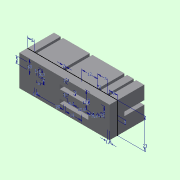
# Autodesk Inventor part: Spirulina_prototype
Saved by Autodesk Inventor 2015 (Build 190159000, 159)
## iProperties
Created: 2015-05-18
Part Number: Spirulina_prototype
Material: Generic
Document SubType Name: Modeling
Designer: Openlab
Density: 1 g/cm^3
Appearance: Default
Author: Openlab
Autodesk Inventor part; units mm, degrees
ref_plane "YZ Plane" through (0, 0, 0) normal (1, 0, 0) x (0, 1, 0)
ref_plane "XZ Plane" through (0, 0, 0) normal (0, 1, 0) x (-1, 0, 0)
ref_plane "XY Plane" through (0, 0, 0) normal (0, 0, 1) x (1, 0, 0)
sketch "Sketch1" plane through (0, 0, 0) normal (0, 1, 0) x (-1, 0, 0)
  line L0 (73.3629, -5.9836) -> (60.8629, -5.9836)
  line L1 (60.8629, -5.9836) -> (60.8629, -18.4836)
  line L2 (60.8629, -18.4836) -> (73.3629, -18.4836)
  line L3 (73.3629, -18.4836) -> (73.3629, -5.9836)
  line L4 (107.9129, -0.7336) -> (40.3129, -0.7336)
  line L5 (40.3129, -23.7336) -> (107.9129, -23.7336)
  line L6 (77.3838, -12.2336) -> (49.3838, -12.2336) construction
  line L7 (67.1129, -2.25) -> (67.1129, -23.25) construction
  line L8 (81.1129, -9.7336) -> (107.9129, -9.7336)
  line L9 (107.9129, -14.7336) -> (81.1129, -14.7336)
  line L10 (48.1129, -23.7336) -> (48.1129, -0.7336)
  line L11 (46.3129, -0.7336) -> (46.3129, -23.7336)
  line L12 (52.6129, -10.7336) -> (40.3129, -10.7336)
  line L13 (52.6129, -13.7336) -> (40.3129, -13.7336)
  line L14 (101.1129, -15.2836) -> (99.6129, -15.2836)
  line L15 (99.6129, -15.2836) -> (99.6129, -9.1836)
  line L16 (99.6129, -9.1836) -> (101.1129, -9.1836)
  line L17 (79.1129, -0.7336) -> (79.1129, -23.7336)
  line L18 (81.1129, -23.7336) -> (81.1129, -0.7336)
  line L19 (55.1129, -0.7336) -> (55.1129, -23.7336)
  line L20 (79.1129, -13.7336) -> (73.3629, -13.7336)
  line L21 (73.3629, -10.7336) -> (79.1129, -10.7336)
  line L22 (60.8629, -13.7336) -> (55.1129, -13.7336)
  line L23 (55.1129, -10.7336) -> (60.8629, -10.7336)
  line L24 (73.3629, -18.4836) -> (77.5629, -18.4836)
  line L25 (77.5629, -18.4836) -> (77.5629, -15.2836)
  line L26 (77.5629, -15.2836) -> (73.3629, -15.2836)
  line L27 (73.3629, -15.2836) -> (60.8629, -15.2836)
  line L28 (56.2629, -15.2836) -> (56.2629, -18.4836)
  line L29 (56.2629, -18.4836) -> (59.4629, -18.4836)
  line L30 (59.4629, -15.2836) -> (56.2629, -15.2836)
  line L31 (59.4629, -5.9836) -> (56.2629, -5.9836)
  line L32 (56.2629, -5.9836) -> (56.2629, -9.1836)
  line L33 (56.2629, -9.1836) -> (59.4629, -9.1836)
  line L34 (60.8629, -9.1836) -> (73.3629, -9.1836)
  line L35 (77.5629, -9.1836) -> (77.5629, -5.9836)
  line L36 (73.3629, -5.9836) -> (77.5629, -5.9836)
  line L37 (77.5629, -9.1836) -> (73.3629, -9.1836)
  line L38 (59.4629, -18.4836) -> (59.4629, -15.2836)
  line L39 (59.4629, -9.1836) -> (59.4629, -5.9836)
  line L40 (60.8629, -18.4836) -> (59.4629, -18.4836)
  line L41 (60.8629, -15.2836) -> (59.4629, -15.2836)
  line L42 (60.8629, -9.1836) -> (59.4629, -9.1836)
  line L43 (60.8629, -5.9836) -> (59.4629, -5.9836)
  line L44 (40.3129, -23.7336) -> (40.3129, -0.7336)
  line L45 (107.9129, -23.7336) -> (107.9129, -0.7336)
  line L46 (53.1129, -14.7336) -> (52.6129, -14.7336)
  line L47 (52.6129, -14.7336) -> (52.6129, -9.7336)
  line L48 (52.6129, -9.7336) -> (53.1129, -9.7336)
  line L49 (53.1129, -23.7336) -> (53.1129, -14.7336)
  line L50 (53.1129, -9.7336) -> (53.1129, -0.7336)
  line L51 (101.1129, -16.2336) -> (98.1129, -16.2336)
  line L52 (98.1129, -16.2336) -> (98.1129, -18.2336)
  line L53 (98.1129, -18.2336) -> (101.1129, -18.2336)
  line L54 (102.9129, -16.2336) -> (105.9129, -16.2336)
  line L55 (105.9129, -16.2336) -> (105.9129, -18.2336)
  line L56 (105.9129, -18.2336) -> (102.9129, -18.2336)
  line L57 (101.1129, -8.2336) -> (98.1129, -8.2336)
  line L58 (98.1129, -8.2336) -> (98.1129, -6.2336)
  line L59 (98.1129, -6.2336) -> (101.1129, -6.2336)
  line L60 (102.9129, -8.2336) -> (105.9129, -8.2336)
  line L61 (105.9129, -8.2336) -> (105.9129, -6.2336)
  line L62 (105.9129, -6.2336) -> (102.9129, -6.2336)
  line L63 (106.4404, -17.2336) -> (97.7013, -17.2336) construction
  line L64 (106, -7.2336) -> (98, -7.2336) construction
  line L65 (102.9129, -23.7336) -> (102.9129, -18.2336)
  line L66 (101.1129, -18.2336) -> (101.1129, -23.7336)
  line L67 (102.9129, -16.2336) -> (102.9129, -8.2336)
  line L68 (102.9129, -6.2336) -> (102.9129, -0.7336)
  line L69 (101.1129, -0.7336) -> (101.1129, -6.2336)
  line L70 (101.1129, -8.2336) -> (101.1129, -16.2336)
  point P0 (102.9129, -9.7336)
  point P1 (101.1129, -9.7336)
  point P2 (102.9129, -14.7336)
  point P3 (101.1129, -14.7336)
  point P4 (48.1129, -10.7336)
  point P5 (46.3129, -10.7336)
  point P6 (48.1129, -13.7336)
  point P7 (46.3129, -13.7336)
  point P8 (67.1129, -12.2336)
  point P9 (99.6129, -9.7336)
  point P10 (99.6129, -14.7336)
  dimension "d0" = 12.5
  dimension "d1" = 12.5
  dimension "d12" = 5
  dimension "d18" = 1.8
  dimension "d39" = 1.5
  dimension "d43" = 2
  dimension "d52" = 12
  dimension "d57" = 12
  dimension "d62" = 3
  dimension "d63" = 3
  dimension "d71" = 7
  dimension "d76" = 4.2
  dimension "d77" = 3.2
  dimension "d78" = 3.2
  dimension "d79" = 1.4
  dimension "d80" = 3.2
  dimension "d91" = 6
  dimension "d92" = 3
  dimension "d95" = 23
  dimension "d98" = 5
  dimension "d99" = 0.5
  dimension "d100" = 2
  dimension "d101" = 2
  dimension "d102" = 3
  dimension "d103" = 10
  dimension "d104" = 1.8
  dimension "d105" = 20
  dimension "d107" = 6.1
  dimension "d108" = 5
  constraints: 138 end point, 56 point on line, 35 perpendicular, 16 vertical, 15 horizontal, 9 collinear, 8 parallel, 4 equal length, 33 other
  measures "d0" distance of L2.end L1.end
  measures "d1" distance of L0.end L1.end
  measures "d12" distance between parallel lines of L9 L8
  measures "d18" distance between parallel lines of L11 L10
  measures "d39" distance of L14.start L14.end
  measures "d43" distance between parallel lines of L18 L17
  measures "d52" distance between parallel lines of L19 L7
  measures "d57" distance between parallel lines of L17 L7
  measures "d62" distance between parallel lines of L21 L20
  measures "d63" distance between parallel lines of L23 L22
  measures "d71" distance between parallel lines of L10 L19
  measures "d76" distance of L2.end L24.end
  measures "d77" distance of L24.end L25.end
  measures "d78" distance of L35.start L35.end
  measures "d79" distance between parallel lines of L38 L1
  measures "d80" distance of L28.end L29.end
  measures "d91" distance between parallel lines of L44 L11
  measures "d92" distance between parallel lines of L12 L13
  measures "d95" distance of L44.start L44.end
  measures "d98" distance of L46.end L47.end
  measures "d99" distance of L46.start L46.end
  measures "d100" distance between parallel lines of L50 L19
  measures "d101" distance of L51.end L52.end
  measures "d102" distance of L52.end L53.end
  measures "d103" distance between parallel lines of L64 L63
  measures "d104" distance between parallel lines of L66 L65
  measures "d105" distance between parallel lines of L18 L66
  measures "d107" distance of L14.end L15.end
  measures "d108" distance between parallel lines of L68 L45
extrude "Extrusion11" add sketch "Sketch1" against normal blind 3 contours L3 L34 L1 L0 | L1 L42 L39 L43 | L3 L2 L1 L27 | L1 L40 L38 L41
extrude "Extrusion10" add sketch "Sketch1" against normal blind 6 separate body contours L0 L43 L31 L32 L33 L42 L1 L23 L19 L4 L17 L21 L3 L37 L35 L36 | L3 L27 L1 L34 | L21 L17 L20 L3 | L1 L22 L19 L23 | L20 L17 L5 L19 L22 L1 L41 L30 L28 L29 L40 L2 L24 L25 L26 L3 | L17 L4 L18 L5 | L19 L5 L49 L46 L47 L48 L50 L4 | L4 L69 L59 L58 L57 L70 L16 L15 L8 L18 | L50 L48 L47 L12 L10 L4 | L18 L9 L15 L14 L70 L51 L52 L53 L66 L5 | L4 L68 L62 L61 L60 L67 L8 L70 L57 L58 L59 L69 | L8 L15 L9 L18 | L5 L10 L13 L47 L46 L49 | L10 L12 L11 L4 | L66 L53 L52 L51 L70 L9 L67 L54 L55 L56 L65 L5 | L4 L45 L8 L67 L60 L61 L62 L68 | L15 L16 L70 L8 | L8 L70 L9 L15 | L5 L11 L13 L10 | L11 L12 L44 L4 | L12 L47 L13 L10 | L10 L13 L11 L12 | L65 L56 L55 L54 L67 L9 L45 L5 | L9 L70 L14 L15 | L8 L67 L9 L70 | L5 L44 L13 L11 | L11 L13 L44 L12 | L45 L9 L67 L8
extrude "Extrusion15" add sketch "Sketch1" along normal blind 5 contours L0 L43 L31 L32 L33 L42 L1 L23 L19 L4 L17 L21 L3 L37 L35 L36 | L21 L17 L20 L3 | L1 L22 L19 L23 | L20 L17 L5 L19 L22 L1 L41 L30 L28 L29 L40 L2 L24 L25 L26 L3 | L4 L69 L59 L58 L57 L70 L16 L15 L8 L18 | L50 L48 L47 L12 L10 L4 | L18 L9 L15 L14 L70 L51 L52 L53 L66 L5 | L8 L15 L9 L18 | L5 L10 L13 L47 L46 L49 | L4 L45 L8 L67 L60 L61 L62 L68 | L15 L16 L70 L8 | L8 L70 L9 L15 | L11 L12 L44 L4 | L12 L47 L13 L10 | L65 L56 L55 L54 L67 L9 L45 L5 | L9 L70 L14 L15 | L5 L44 L13 L11 | L11 L13 L44 L12 | L45 L9 L67 L8
extrude "Extrusion14" add sketch "Sketch1" along normal blind 3.5 contours L3 L34 L1 L0 | L3 L27 L1 L34 | L3 L2 L1 L27
extrude "Extrusion16" add sketch "Sketch1" along normal blind 20 contours L0 L43 L31 L32 L33 L42 L1 L23 L19 L4 L17 L21 L3 L37 L35 L36 | L1 L42 L39 L43 | L20 L17 L5 L19 L22 L1 L41 L30 L28 L29 L40 L2 L24 L25 L26 L3 | L1 L40 L38 L41 | L4 L69 L59 L58 L57 L70 L16 L15 L8 L18 | L50 L48 L47 L12 L10 L4 | L18 L9 L15 L14 L70 L51 L52 L53 L66 L5 | L5 L10 L13 L47 L46 L49 | L4 L45 L8 L67 L60 L61 L62 L68 | L11 L12 L44 L4 | L65 L56 L55 L54 L67 L9 L45 L5 | L5 L44 L13 L11
body "Solid3"
